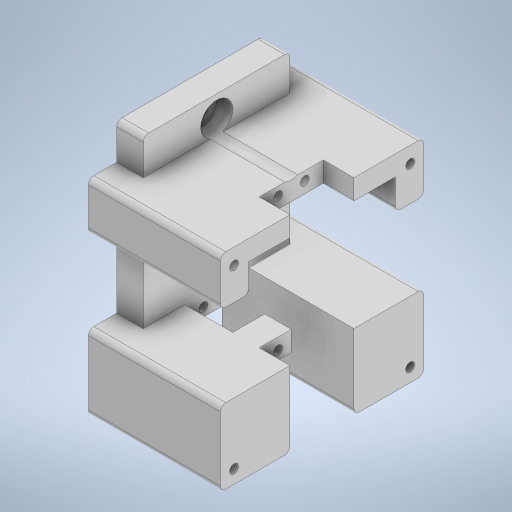
# Autodesk Inventor part: separator_plate_alternate
Saved by Autodesk Inventor 2023 (Build 270158000, 158)
## iProperties
Created: 2023-01-24
Part Number: separator_plate_alternate
Material: Generic
Document SubType Name: Modeling
Designer: Hunter
Density: 1 g/cm^3
Appearance: Default
Author: Hunter
Autodesk Inventor part; units mm, degrees
ref_plane "YZ Plane" through (0, 0, 0) normal (1, 0, 0) x (0, 1, 0)
ref_plane "XZ Plane" through (0, 0, 0) normal (0, 1, 0) x (-1, 0, 0)
ref_plane "XY Plane" through (0, 0, 0) normal (0, 0, 1) x (1, 0, 0)
sketch "Sketch1" plane through (0, 0, 0) normal (1, 0, 0) x (0, 1, 0)
  line L0 (0, 27.5) -> (-57, 27.5)
  line L1 (-57, -27.5) -> (0, -27.5)
  line L2 (0, -27.5) -> (0, 27.5)
  line L3 (0, 0) -> (-57, 0) construction
  circle A0 centre (-38.25, 15) radius 3
  circle A1 centre (-38.25, -15) radius 3
  circle A2 centre (-8, 0) radius 3
  line L4 (-57, 27.5) -> (-70, 27.5)
  line L5 (-70, 27.5) -> (-70, -27.5)
  line L6 (-70, -27.5) -> (-57, -27.5)
  point P0 (-29.3628, 0)
  dimension "d0" = 55
  dimension "d1" = 57
  dimension "d103" = 8
  dimension "d104" = 27.5
  dimension "d129" = 30
  dimension "d130" = 30.25
  dimension "d131" = 13
  dimension "d132" = 55
  dimension "d133" = 6
  dimension "d134" = 6
  dimension "d135" = 6
  constraints: 14 end point, 3 centre point, 2 horizontal, 2 perpendicular, 1 coincident, 1 midpoint, 1 parallel, 1 point on line
  measures "d0" distance of L1.end L0.start
  measures "d1" distance of L0.start L0.end
  measures "d103" distance from line of L2 A2.centre
  measures "d104" distance from line of L1 A2.centre
  measures "d129" distance of A0.centre A1.centre
  measures "d130" horizontal distance of A1.centre A2.centre
  measures "d131" distance of L0.end L4.end
  measures "d132" distance of L4.end L5.end
  measures "d133" diameter of A1
  measures "d134" diameter of A0
  measures "d135" diameter of A2
extrude "Extrusion1" add sketch "Sketch1" along normal blind 10
sketch "Sketch2" plane through (10, 0, 0) normal (1, 0, 0) x (0, 0, -1)
  line L0 (-27.5, 0) -> (-27.5, -70) projected
  line L1 (-27.5, -21) -> (27.5, -21)
  line L2 (27.5, 0) -> (-27.5, 0) projected
  line L3 (-27.5, -13.5) -> (27.5, -13.5)
  line L4 (27.5, -70) -> (27.5, 0) projected
  line L5 (-27.5, -62.5) -> (27.5, -62.5)
  line L6 (-27.5, -70) -> (27.5, -70) projected
  line L7 (-27.5, -70) -> (27.5, -70)
  line L8 (27.5, -70) -> (27.5, -62.5)
  line L9 (-27.5, -70) -> (-27.5, -62.5)
  dimension "d139" = 21
  dimension "d140" = 7.5
  dimension "d141" = 7.5
  constraints: 12 end point, 5 point on line, 3 horizontal, 2 collinear, 1 parallel
  measures "d139" distance between parallel lines of L1 L2
  measures "d140" distance between parallel lines of L1 L3
  measures "d141" distance between parallel lines of L6 L5
extrude "Extrusion8" add sketch "Sketch2" along normal blind 28 contours L3 L4 L1 L0 | L5 L4 L6 L0
sketch "Sketch10" plane through (38, 0, 0) normal (1, 0, 0) x (0, 0, -1)
  circle A0 centre (-5, -66.75) radius 1.65
  circle A1 centre (5, -66.75) radius 1.65
  line L0 (27.5, -13.5) -> (-27.5, -13.5) projected
  circle A2 centre (-5, -16.75) radius 1.65
  circle A3 centre (5, -16.75) radius 1.65
  line L1 (-27.5, -21) -> (27.5, -21) projected
  line L2 (-5, -66.75) -> (5, -66.75) construction
  line L3 (-27.5, -62.5) -> (-27.5, -70) construction
  point P0 (0, 0)
  point P1 (0, -66.75)
  dimension "d79" = 10
  dimension "d144" = 3.3
  dimension "d145" = 3.3
  dimension "d146" = 10
  dimension "d147" = 4.25
  dimension "d148" = 50
  constraints: 4 centre point, 2 end point, 2 equal radius, 2 horizontal alignment, 2 vertical alignment, 1 horizontal, 1 midpoint
  measures "d79" distance of L2.end L2.start
  measures "d144" diameter of A1
  measures "d145" diameter of A0
  measures "d146" distance of A3.centre A2.centre
  measures "d147" distance from line of L1 A2.centre
  measures "d148" distance of L2.start A2.centre
sketch "Sketch14" plane through (38, 0, 0) normal (1, 0, 0) x (0, 0, -1)
  circle A0 centre (-15, -38.25) radius 3 construction
  circle A1 centre (-15, -38.25) radius 3 construction
  circle A2 centre (-15, -38.25) radius 6
  circle A3 centre (15, -38.25) radius 3 construction
  circle A4 centre (15, -38.25) radius 6
  circle A5 centre (0, -8) radius 3 construction
  circle A6 centre (0, -8) radius 6
  point P0 (0, 0)
  point P1 (-15, -35.25)
  point P2 (-15, -35.25)
  point P3 (15, -35.25)
  point P4 (15, -35.25)
  point P5 (-15, -35.25)
  point P6 (15, -35.25)
  dimension "d108" = 12
  dimension "d109" = 12
  dimension "d112" = 12
  constraints: 3 centre point, 3 coincident
  measures "d108" diameter of A2
  measures "d109" diameter of A4
  measures "d112" diameter of A6
sketch "Sketch15" plane through (38, 0, 0) normal (1, 0, 0) x (0, 0, -1)
  line L0 (-38.1, -90.6) -> (38.1, -90.6)
  line L1 (27.5, -81) -> (-27.5, -81)
  line L2 (-38.1, -14.4) -> (-38.1, -24)
  line L3 (-38.1, -81) -> (-38.1, -90.6)
  line L4 (38.1, -90.6) -> (38.1, -73.5)
  line L5 (38.1, -24) -> (38.1, -14.4)
  line L6 (-12, -90.6) -> (-12, -81)
  line L7 (12, -90.6) -> (12, -81)
  line L8 (-38.1, -73.5) -> (-38.1, -81)
  line L9 (-38.1, -31.5) -> (-38.1, -24)
  line L10 (27.5, -62.5) -> (-27.5, -62.5) projected
  line L11 (-38.1, -14.4) -> (38.1, -14.4)
  line L12 (-38.1, -73.5) -> (-27.5, -73.5)
  line L13 (27.5, -81) -> (27.5, -73.5)
  line L14 (27.5, -62.5) -> (27.5, -21) projected
  line L15 (-27.5, -73.5) -> (-27.5, -81)
  line L16 (27.5, -73.5) -> (38.1, -73.5)
  line L17 (-38.1, -31.5) -> (-27.5, -31.5)
  line L18 (-27.5, -31.5) -> (-27.5, -24)
  line L19 (38.1, -24) -> (38.1, -32.5)
  line L20 (38.1, -32.5) -> (27.5, -32.5)
  line L21 (27.5, -25) -> (27.5, -32.5)
  line L22 (-12, -21) -> (-12, -13.5)
  line L23 (12, -21) -> (12, -13.5)
  circle A0 centre (-33.02, -85.52) radius 1.65
  circle A1 centre (-33.02, -19.48) radius 1.65
  circle A2 centre (33.02, -19.48) radius 1.65
  circle A3 centre (33.02, -85.52) radius 1.65
  line L24 (-38.1, -14.4) -> (38.1, -14.4)
  line L25 (-27.5, -24) -> (-27.5, -21)
  line L26 (-27.5, -21) -> (27.5, -21) projected
  line L27 (27.5, -21) -> (27.5, -25)
  line L28 (-12, -81) -> (-27.5, -81)
  line L29 (-38.1, -81.6423) -> (-38.1, -62.5)
  line L30 (-38.1, -62.5) -> (-12, -62.5)
  line L31 (-12, -62.5) -> (-12, -81)
  line L32 (12, -81) -> (27.5, -81)
  line L33 (38.1, -81.6423) -> (38.1, -62.5)
  line L34 (38.1, -62.5) -> (12, -62.5)
  line L35 (12, -62.5) -> (12, -81)
  line L36 (-5, -66.75) -> (5, -66.75) construction
  line L37 (0, -52.5) -> (0, -66.75) construction
  line L38 (-38.1, -14.4) -> (38.1, -14.4)
  line L39 (38.1, -14.4) -> (38.1, -13.5)
  line L40 (12, -13.5) -> (38.1, -13.5)
  circle A4 centre (0, -52.5) radius 10 construction
  line L41 (-12, -13.5) -> (-38.1, -13.5)
  line L42 (-38.1, -13.5) -> (-38.1, -14.4)
  line L43 (-38.1, -14.4) -> (-12, -14.4)
  line L44 (-12, -14.4) -> (-12, -13.5)
  point P0 (0, -81)
  point P1 (27.5, 0)
  point P2 (12, -57)
  point P3 (-12, -57)
  point P4 (-88.499, -121.9266)
  point P5 (12, -14.4)
  point P6 (12, -85.8)
  point P7 (38.1, -73.5)
  point P8 (12, -62.5)
  point P9 (-12, -62.5)
  point P10 (-38.1, -73.5)
  point P11 (38.1, -19.2)
  point P12 (38.1, -14.4)
  point P13 (12, -14.4)
  dimension "d121" = 76.2
  dimension "d122" = 7
  dimension "d123" = 7
  dimension "d154" = 9.6
  dimension "d162" = 9.6
  dimension "d164" = 38.1
  dimension "d165" = 7.5
  dimension "d166" = 9.6
  dimension "d168" = 10.6
  dimension "d169" = 0
  dimension "d170" = 17.1
  dimension "d171" = 38.1
  dimension "d173" = 7.5
  dimension "d174" = 7.5
  dimension "d175" = 9.6
  dimension "d176" = 7.5
  dimension "d177" = 10.6
  dimension "d178" = 10.6
  dimension "d179" = 5.08
  dimension "d180" = 5.08
  dimension "d181" = 5.08
  dimension "d202" = 3.3
  dimension "d204" = 4.25
  dimension "d205" = 20
  dimension "d206" = 76.2
  dimension "d208" = 7.5
  dimension "d209" = 7.5
  constraints: 84 end point, 14 point on line, 13 perpendicular, 11 parallel, 9 horizontal, 5 centre point, 5 vertical, 4 midpoint, 3 equal radius, 2 horizontal alignment, 2 vertical alignment, 1 coincident, 1 collinear, 1 tangent
  measures "d121" distance of L0.start L0.end
  measures "d122" distance from line of L36.start L6
  measures "d123" distance from line of L7 L36.end
  measures "d154" distance between parallel lines of L0 L1
  measures "d162" distance of L5.start L5.end
  measures "d164" distance from line of L37.start L0
  measures "d165" distance of L8.start L3.start
  measures "d166" distance of L3.start L0.start
  measures "d168" distance of L8.start L12.end
  measures "d169" distance between parallel lines of L12 L16
  measures "d170" distance of L0.end L4.end
  measures "d171" distance from line of L37.start L11
  measures "d173" distance of L17.end L18.end
  measures "d174" distance of L21.start L20.end
  measures "d175" distance of L2.start L2.end
  measures "d176" distance of L9.start L2.end
  measures "d177" distance of L9.start L17.end
  measures "d178" distance of L19.end L20.end
  measures "d179" distance from line of L11 A1.centre
  measures "d180" distance from line of L2 A1.centre
  measures "d181" distance from line of L0 A0.centre
  measures "d202" diameter of A1
  measures "d204" distance from line of L10 L36.start
  measures "d205" diameter of A4
  measures "d206" distance of L2.start L24.end
  measures "d208" distance of L22.start L22.end
  measures "d209" distance of L23.start L23.end
extrude "Extrusion17" add sketch "Sketch15" against normal up to surface (38 mm away) contours L1 L15 L12 L29 L30 L10 L31 | L35 L10 L34 L33 L16 L13 L1
extrude "Extrusion18" add sketch "Sketch15" along normal blind 11.5 and the other way blind 38 contours L3 L8 L12 L15 L1 L6 L0 | L7 L1 L13 L16 L4 L0 | L1 L15 L12 L29 L30 L10 L31 | L35 L10 L34 L33 L16 L13 L1 | L11 L22 L26 L25 L18 L17 L9 L2 | L42 L41 L22 L11 | L23 L40 L39 L11 | L11 L5 L19 L20 L14 L26 L23
extrude "Extrusion19" cut sketch "Sketch10" against normal through all
extrude "Extrusion20" cut sketch "Sketch14" against normal blind 34
sketch "Sketch16" plane through (38, 0, 0) normal (1, 0, 0) x (0, 0, -1)
  line L0 (-12, -70) -> (12, -70) projected
  line L1 (12, -70) -> (12, -62.5)
  line L2 (-27.5, -62.5) -> (27.5, -62.5) projected
  line L3 (-12, -70) -> (12, -70) projected
  line L4 (0, -70) -> (0, -62.5)
  point P0 (0, 0)
  point P1 (27.5, -70)
  point P2 (-27.5, -70)
  point P3 (12, -66.25)
  dimension "d191" = 12
  constraints: 4 end point, 2 midpoint, 2 vertical, 1 point on line
  measures "d191" distance from line of point (12, -66.25) L4
extrude "Extrusion21" cut sketch "Sketch16" against normal blind 28
sketch "Sketch18" plane through (0, -70, -12) normal (0, -1, 0) x (1, 0, 0)
  line L0 (10, -15.5) -> (10, 39.5) projected
  line L1 (10, 12) -> (28, 12)
  line L2 (28, 12) -> (28, 24)
  line L3 (28, 24) -> (10, 24)
  line L4 (10, 24) -> (10, 12)
  line L5 (38, 24) -> (38, 12) projected
  point P0 (0, 12)
  dimension "d197" = 10
  dimension "d198" = 12
  constraints: 8 end point, 2 parallel, 1 horizontal, 1 midpoint, 1 perpendicular
  measures "d197" distance between parallel lines of L2 L5
  measures "d198" distance of L1.end L2.end
extrude "Extrusion23" cut sketch "Sketch18" against normal blind 9
fillet "Fillet9" radius 2 12 edges at (24.75, -32.5, -38.1) (29.75, -32.5, -27.5) (29.75, -31.5, 27.5) (24.75, -31.5, 38.1) (24.75, -90.6, 38.1) (24.75, -62.5, 38.1) (24.75, -90.6, 12) (24.75, -90.6, -12) (24.75, -90.6, -38.1) (24.75, -62.5, -38.1) (5, 0, 27.5) (5, 0, -27.5)
fillet "Fillet10" radius 2 2 edges at (24.75, -13.5, 38.1) (24.75, -13.5, -38.1)
body "Solid1"
